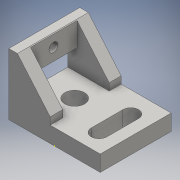
# Autodesk Inventor part: 240510_3Dsketch05
Saved by Autodesk Inventor 2016 (Build 200138000, 138)
## iProperties
Created: 2024-05-10
Part Number: 240510_3Dsketch05
Material: 일반
Document SubType Name: Modeling
Designer: pc
Density: 1 g/cm^3
Appearance: 기본값
Author: pc
Autodesk Inventor part; units mm, degrees
ref_plane "YZ Plane" through (0, 0, 0) normal (1, 0, 0) x (0, 1, 0)
ref_plane "XZ Plane" through (0, 0, 0) normal (0, 1, 0) x (-1, 0, 0)
ref_plane "XY Plane" through (0, 0, 0) normal (0, 0, 1) x (1, 0, 0)
sketch "스케치1" plane through (0, 0, 0) normal (0, 0, 1) x (1, 0, 0)
  line L0 (20.0206, -15.5449) -> (-20.0206, -15.5449)
  line L1 (-20.0206, -15.5449) -> (-20.0206, 15.5449)
  line L2 (-20.0206, 15.5449) -> (20.0206, 15.5449)
  line L3 (20.0206, 15.5449) -> (20.0206, -15.5449)
  line L4 (20.0206, -15.5449) -> (-20.0206, 15.5449) construction
  line L5 (-20.0206, -15.5449) -> (20.0206, 15.5449) construction
  point P0 (0, 0)
  constraints: 12 end point, 2 midpoint, 2 parallel, 1 horizontal, 1 perpendicular
extrude "돌출1" add sketch "스케치1" along normal blind 7
sketch "스케치2" plane through (0, 0, 7) normal (0, 0, 1) x (1, 0, 0)
  line L0 (20.0206, 15.5449) -> (-20.0206, 15.5449) projected
  line L1 (-20.0206, -15.5449) -> (20.0206, -15.5449) projected
  line L2 (-20.0206, 15.5449) -> (-1.902, 15.5449)
  line L3 (-1.902, 15.5449) -> (-1.902, -15.5449)
  line L4 (-1.902, -15.5449) -> (-20.0206, -15.5449)
  line L5 (-20.0206, -15.5449) -> (-20.0206, 15.5449)
  point P0 (0, 0)
  constraints: 8 end point, 2 parallel, 1 horizontal, 1 perpendicular, 1 point on line
extrude "돌출2" add sketch "스케치2" along normal blind 20
sketch "스케치3" plane through (-20.0206, -15.5449, 0) normal (0, -1, 0) x (1, 0, 0)
  point P0 (20.0206, 0)
sketch "스케치4" plane through (-20.0206, -15.5449, 0) normal (0, -1, 0) x (1, 0, 0)
  point P0 (20.0206, 0)
sketch "스케치5" plane through (0, 0, 27) normal (0, 0, 1) x (1, 0, 0)
  line L0 (-1.902, -15.5449) -> (-1.902, 15.5449) projected
  line L1 (-1.902, -10.0538) -> (-16.0103, -10.0538)
  line L2 (-16.0103, -10.0538) -> (-16.0103, 10.3292)
  line L3 (-16.0103, 10.3292) -> (-1.902, 10.3292)
  point P0 (0, 0)
  constraints: 6 end point, 2 perpendicular, 2 point on line, 1 horizontal
extrude "돌출3" cut sketch "스케치5" against normal blind 20
sketch "스케치6" plane through (-20.0206, -15.5449, 0) normal (0, -1, 0) x (1, 0, 0)
  line L0 (3.8381, 26.8904) -> (18.1186, 10.1571)
  line L1 (18.1186, 7) -> (18.1186, 27) projected
  point P0 (20.0206, 0)
  constraints: 2 end point, 1 point on line
extrude "돌출4" cut sketch "스케치6" against normal blind 50 fills toward (11.0164, 18.5562) open curves L0
sketch "스케치7" plane through (-16.0103, -10.0538, 7) normal (1, 0, 0) x (0, 0, -1)
  point P0 (7, 10.0538)
sketch "스케치8" plane through (-20.0206, -15.5449, 0) normal (-1, 0, 0) x (0, 0, 1)
  line L0 (7, 5.4911) -> (10.1571, 5.4911) projected
  line L1 (26.6887, 25.8742) -> (7, 25.8742) projected
  line L2 (7, 5.4911) -> (16.3344, 5.4911)
  line L3 (16.3344, 5.4911) -> (16.3344, 25.8742)
  line L4 (16.3344, 25.8742) -> (7, 25.8742)
  line L5 (7, 25.8742) -> (7, 5.4911)
  point P0 (0, 15.5449)
  constraints: 8 end point, 2 parallel, 1 horizontal, 1 perpendicular, 1 point on line
extrude "돌출5" cut sketch "스케치8" against normal blind 50
sketch "스케치9" plane through (0, 0, 7) normal (0, 0, 1) x (1, 0, 0)
  circle A0 centre (-6.706, 0) radius 4.3291
  arc A1 (14.9835, 6.3061) -> (8.1492, 6.3061) centre (11.5664, 6.3061) ccw
  arc A2 (8.1492, -7.5981) -> (14.9835, -7.5981) centre (11.5664, -7.5981) ccw
  line L0 (8.1492, 6.3061) -> (8.1492, -7.5981)
  line L1 (14.9835, 6.3061) -> (14.9835, -7.5981)
  point P0 (0, 0)
  constraints: 4 end point, 4 point on circle, 3 centre point, 1 tangent, 1 vertical
extrude "돌출6" cut sketch "스케치9" against normal blind 50
sketch "스케치10" plane through (-16.0103, -10.0538, 26.6887) normal (1, 0, 0) x (0, 0, -1)
  circle A0 centre (4.971, 10.0538) radius 1.9853
  point P0 (26.6887, 10.0538)
  constraints: 1 centre point
extrude "돌출7" cut sketch "스케치10" against normal blind 50
